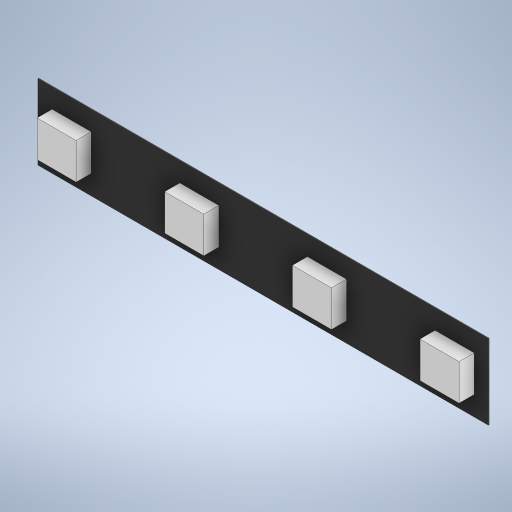
# Autodesk Inventor part: 네오픽셀
Saved by Autodesk Inventor 2023 (Build 270158000, 158)
## iProperties
Created: 2022-11-10
Part Number: 네오픽셀
Material: 일반
Document SubType Name: Modeling
Designer: user
Density: 1 g/cm^3
Appearance: 기본값
Author: user
Autodesk Inventor part; units mm, degrees
ref_plane "YZ Plane" through (0, 0, 0) normal (1, 0, 0) x (0, 1, 0)
ref_plane "XZ Plane" through (0, 0, 0) normal (0, 1, 0) x (-1, 0, 0)
ref_plane "XY Plane" through (0, 0, 0) normal (0, 0, 1) x (1, 0, 0)
sketch "스케치1" plane through (0, 0, 0) normal (0, 0, 1) x (1, 0, 0)
  line L0 (-30, 5) -> (30, 5)
  line L1 (30, 5) -> (30, -5)
  line L2 (30, -5) -> (-30, -5)
  line L3 (-30, -5) -> (-30, 5)
  line L4 (-30, 5) -> (30, -5) construction
  line L5 (30, 5) -> (-30, -5) construction
  point P0 (0, 0)
  dimension "d0" = 60
  dimension "d1" = 10
  constraints: 12 end point, 2 midpoint, 2 parallel, 1 horizontal, 1 perpendicular
  measures "d0" distance of L1.end L2.end
  measures "d1" distance of L0.end L1.end
extrude "돌출1" add sketch "스케치1" along normal blind 0.1
sketch "스케치2" plane through (0, 0, 0.1) normal (0, 0, 1) x (1, 0, 0)
  line L0 (-28.1, -2.4) -> (-22.9, -2.4)
  line L1 (-22.9, -2.4) -> (-22.9, 2.4)
  line L2 (-22.9, 2.4) -> (-28.1, 2.4)
  line L3 (-28.1, 2.4) -> (-28.1, -2.4)
  line L4 (-28.1, -2.4) -> (-22.9, 2.4) construction
  line L5 (-22.9, -2.4) -> (-28.1, 2.4) construction
  line L6 (-30, 5) -> (-30, -5) projected
  line L7 (-11.1, -2.4) -> (-5.9, -2.4)
  line L8 (-5.9, -2.4) -> (-5.9, 2.4)
  line L9 (-5.9, 2.4) -> (-11.1, 2.4)
  line L10 (-11.1, 2.4) -> (-11.1, -2.4)
  line L11 (-11.1, -2.4) -> (-5.9, 2.4) construction
  line L12 (-5.9, -2.4) -> (-11.1, 2.4) construction
  line L13 (5.9, -2.4) -> (11.1, -2.4)
  line L14 (11.1, -2.4) -> (11.1, 2.4)
  line L15 (11.1, 2.4) -> (5.9, 2.4)
  line L16 (5.9, 2.4) -> (5.9, -2.4)
  line L17 (5.9, -2.4) -> (11.1, 2.4) construction
  line L18 (11.1, -2.4) -> (5.9, 2.4) construction
  line L19 (22.9, -2.4) -> (28.1, -2.4)
  line L20 (28.1, -2.4) -> (28.1, 2.4)
  line L21 (28.1, 2.4) -> (22.9, 2.4)
  line L22 (22.9, 2.4) -> (22.9, -2.4)
  line L23 (22.9, -2.4) -> (28.1, 2.4) construction
  line L24 (28.1, -2.4) -> (22.9, 2.4) construction
  line L25 (-5.9, 0) -> (5.9, 0)
  point P0 (0, 0)
  point P1 (-25.5, 0)
  point P2 (-8.5, 0)
  point P3 (8.5, 0)
  point P4 (25.5, 0)
  point P5 (0, 0)
  dimension "d4" = 5.2
  dimension "d5" = 4.8
  dimension "d9" = 17
  constraints: 50 end point, 5 midpoint, 2 horizontal, 2 parallel, 1 coincident, 1 collinear, 1 horizontal alignment, 1 perpendicular, 32 other
  measures "d4" distance of L2.end L1.end
  measures "d5" distance of L1.end L0.end
  measures "d9" distance of L0.start L7.start
extrude "돌출2" add sketch "스케치2" along normal blind 2
